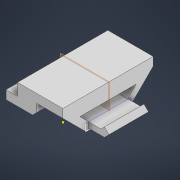
# Autodesk Inventor part: FRC Pit Hook
Saved by Autodesk Inventor 2022 (Build 260153000, 153)
## iProperties
Created: 2021-10-08
Part Number: FRC Pit Hook
Material: Generic
Document SubType Name: Modeling
Designer: izack
Density: 1 g/cm^3
Appearance: Default
Author: izack
Autodesk Inventor part; units mm, degrees
ref_plane "YZ Plane" through (0, 0, 0) normal (1, 0, 0) x (0, 1, 0)
ref_plane "XZ Plane" through (0, 0, 0) normal (0, 1, 0) x (-1, 0, 0)
ref_plane "XY Plane" through (0, 0, 0) normal (0, 0, 1) x (1, 0, 0)
sketch "Sketch1" plane through (0, 0, 0) normal (0, 1, 0) x (-1, 0, 0)
  line L0 (0, 0) -> (13.97, 0)
  line L1 (13.97, 0) -> (13.97, -15.748)
  line L2 (13.97, -15.748) -> (0, -15.748)
  line L3 (0, -15.748) -> (0, 0)
  line L4 (13.97, -49.53) -> (0, -49.53)
  line L5 (0, -49.53) -> (0, -65.278)
  line L6 (0, -65.278) -> (13.97, -65.278)
  line L7 (13.97, -65.278) -> (13.97, -49.53)
  dimension "d0" = 13.97
  dimension "d1" = 15.748
  dimension "d2" = 15.748
  dimension "d3" = 33.782
  constraints: 16 end point, 4 parallel, 2 horizontal, 2 perpendicular, 2 point on line
  measures "d0" distance of L1.end L2.end
  measures "d1" distance of L0.end L1.end
  measures "d2" distance of L5.end L4.end
  measures "d3" distance between parallel lines of L2 L4
extrude "Extrusion1" add sketch "Sketch1" along normal blind 2.286
sketch "Sketch2" plane through (0, 2.286, 0) normal (0, 1, 0) x (1, 0, 0)
  line L0 (-13.97, 15.748) -> (-13.97, 0) projected
  line L1 (-13.97, 0) -> (0, 0)
  line L2 (0, 0) -> (0, 65.278)
  line L3 (0, 65.278) -> (-13.97, 65.278)
  line L4 (-13.97, 65.278) -> (-13.97, 0)
  point P0 (0, 0)
  constraints: 8 end point, 2 parallel, 1 horizontal, 1 perpendicular
extrude "Extrusion2" add sketch "Sketch2" along normal blind 6.35
sketch "Sketch3" plane through (0, 0, -49.53) normal (1, 0, 0) x (0, 0, -1)
  line L0 (-49.53, 8.636) -> (15.748, 8.636) projected
  line L1 (15.748, 0) -> (15.748, 8.636) projected
  line L2 (-49.53, 8.636) -> (15.748, 8.636)
  line L3 (15.748, 8.636) -> (15.748, 2.5059)
  line L4 (15.748, 2.5059) -> (-49.53, 2.5059)
  line L5 (-49.53, 2.5059) -> (-49.53, 8.636)
  point P0 (-49.53, 0)
  constraints: 8 end point, 2 parallel, 1 horizontal, 1 perpendicular, 1 point on line
extrude "Extrusion3" add sketch "Sketch3" along normal blind 12.446
sketch "Sketch4" plane through (12.446, 0, -49.53) normal (1, 0, 0) x (0, 0, -1)
  line L0 (15.748, 8.636) -> (-49.53, 8.636) projected
  line L1 (-49.53, 8.636) -> (15.748, 8.636)
  line L2 (15.748, 8.636) -> (15.748, 2.5059)
  line L3 (15.748, 2.5059) -> (-49.53, 2.5059)
  line L4 (-49.53, 0) -> (-49.53, 8.636) projected
  line L5 (-49.53, 8.636) -> (-49.53, 2.5059)
  line L6 (-49.53, 2.5059) -> (-24.0466, 2.5059) construction
  line L7 (-16.891, 8.636) -> (-16.891, -118.364) construction
  line L8 (15.748, 2.5059) -> (-49.53, 2.5059) projected
  line L9 (-49.53, 2.5059) -> (-16.891, -30.1331)
  line L10 (-49.53, 2.5059) -> (-3.3715, 2.5059) construction
  line L11 (-16.891, -30.1331) -> (15.748, 2.5059)
  line L12 (-33.2105, -13.8136) -> (-0.5715, -13.8136)
  line L13 (-16.891, -8.7336) -> (-2.6757, -8.7336)
  line L14 (-49.53, 2.5059) -> (15.748, 2.5059) projected
  line L15 (-2.6757, -8.7336) -> (3.4838, -2.5741)
  line L16 (3.4838, -2.5741) -> (-36.2655, -2.5741)
  line L17 (-30.106, -8.7336) -> (-16.891, -8.7336)
  line L18 (-16.891, -8.7336) -> (-31.1063, -8.7336)
  line L19 (-31.1063, -8.7336) -> (-37.2658, -2.5741)
  line L20 (-37.2658, -2.5741) -> (2.4835, -2.5741)
  point P0 (-30.106, -8.7336)
  point P1 (-36.2655, -2.5741)
  dimension "d13" = 127
  dimension "d14" = 45
  dimension "d15" = 5.08
  dimension "d16" = 5.08
  dimension "d17" = 5.08
  constraints: 34 end point, 5 perpendicular, 4 point on line, 3 horizontal, 3 midpoint, 3 symmetric about line, 2 parallel, 1 collinear, 1 equal length, 1 vertical
  measures "d13" distance of L7.start L7.end
  measures "d14" angle of L9 L10
  measures "d15" distance between parallel lines of L12 L13
  measures "d16" distance between parallel lines of L11 L15
  measures "d17" distance between parallel lines of L10 L16
extrude "Extrusion4" add sketch "Sketch4" along normal blind 6.35 contours L2 L3 L4 L0 | L11 L12 L9 L3
sketch "Sketch5" plane through (18.796, 0, -49.53) normal (1, 0, 0) x (0, 0, -1)
  line L0 (-33.2105, -13.8136) -> (-0.5715, -13.8136) projected
  line L1 (-33.2105, -13.8136) -> (-0.5715, -13.8136)
  line L2 (-0.5715, -13.8136) -> (-0.5715, -8.8161)
  line L3 (-0.5715, -8.8161) -> (-33.2105, -8.8161)
  line L4 (-33.2105, -8.8161) -> (-33.2105, -13.8136)
  point P0 (-49.53, 0)
  constraints: 8 end point, 2 parallel, 1 horizontal, 1 perpendicular
ref_plane "Work Plane1" through (-13.97, 0, -32.639) normal (0, 0, 1) x (1, 0, 0)
sketch "Sketch6" plane through (-13.97, 0, -32.639) normal (0, 0, 1) x (1, 0, 0)
  line L0 (26.416, -8.7336) -> (32.766, -8.7336) projected
  line L1 (32.766, -8.7336) -> (41.9683, -8.7336)
  line L2 (41.9683, -8.7336) -> (44.4776, -6.1913)
  line L3 (44.4776, -6.1913) -> (47.7281, -9.3996)
  line L4 (47.7281, -9.3996) -> (44.4776, -12.6928)
  line L5 (44.4776, -12.6928) -> (32.766, -12.6928)
  line L6 (32.766, -8.7336) -> (32.766, -12.6928)
  line L7 (32.766, 2.5059) -> (32.766, -13.8136) projected
  point P0 (13.97, 0)
  constraints: 12 end point, 1 collinear, 1 horizontal, 1 parallel, 1 perpendicular
extrude "Extrusion5" add sketch "Sketch6" along normal mid plane 28.575
sketch "Sketch7" plane through (0, 0, 0) normal (0, -1, 0) x (1, 0, 0)
  line L0 (0, -65.278) -> (0, 0) projected
  line L1 (0, -65.278) -> (-22.225, -65.278)
  line L2 (-22.225, -65.278) -> (-22.225, -49.53)
  line L3 (-22.225, -49.53) -> (0, -49.53)
  line L4 (0, -49.53) -> (0, -65.278)
  line L5 (-13.97, -65.278) -> (-13.97, 0) construction
  line L6 (-13.97, -32.639) -> (9.5461, -32.639) construction
  line L7 (0, 0) -> (0, -65.278)
  line L8 (0, 0) -> (-22.225, 0)
  line L9 (-22.225, 0) -> (-22.225, -15.748)
  line L10 (-22.225, -15.748) -> (0, -15.748)
  point P0 (0, -49.53)
  point P1 (0, -15.748)
  dimension "d24" = 22.225
  constraints: 18 end point, 5 symmetric about line, 2 horizontal, 2 parallel, 1 midpoint, 1 perpendicular
  measures "d24" distance of L2.end L3.end
extrude "Extrusion6" add sketch "Sketch7" along normal blind 6.35
chamfer "Chamfer1" distance 3.175 angle 45 2 edges at (0, -6.35, -7.874) (0, -6.35, -57.404)
chamfer "Chamfer2" distance 1.0795 angle 45 1 edges at (18.796, -12.6928, -32.639)
body "Solid1"
